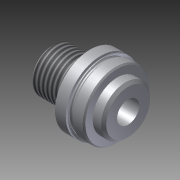
# Autodesk Inventor part: 04000_rod_guide
Saved by Autodesk Inventor 2012 (Build 160160000, 160)
## iProperties
Category: PARTsolutions
Company: BIMBA
Created: 2013-01-17
Part Number: 04000_rod_guide
Material: Default
Catalog Web Link: www.cadenas.de
Description: Rod Guide-Original Line - Standard Air Cylinders
Vendor: BIMBA
Document SubType Name: Modeling
Designer: William
Manufacturer: BIMBA
Density: 1 g/cm^3
Mass: 3.5706 g
Surface Area: 22.4703 cm^2
Volume: 3.5706 cm^3
PSOL_IDENT_0: {\\10.0.0.242\data_v9\23d-libs\bimba\bimba\bimba_imperial\bimba_full_line\original_line_cylinders\st
PSOL_IDENT_1: andard_air_cylinders\rod_guide.prj},217 {VTYP=3D},{NB=04000_rod_guide},{LINA=04000_rod_guide},{NN=Ro
PSOL_IDENT_2: d Guide},{DATE=11.09.2012 04:45:35},{GEOMDATE=11.09.2012 04:45:00},{VERSION=},{LINEID=40},{LINESUBID
PSOL_IDENT_3: =-1},{WBVAR=MNT,ACTING,NR,K,Q,T1,T2,T3,T4,MB,TRIM,CUSH}  {NB=04000_rod_guide},{LINA=04000_rod_guide}
PSOL_IDENT_4: ,{KT=DUMMY},{PN=04000},{BORE=0.75000000},{BOREPN=04},{MNT=},{MNTALG='' , 'Front Nose' , 'BF' , 'Fron
PSOL_IDENT_5: t Block' , 'BFT' , 'Front Trunnion' , 'A' , 'Adjustable Stroke'},{ACTING=},{ACTINGALG= '' , 'Single
PSOL_IDENT_6: Acting' , 'R' , 'Reverse/Double Acting' },{NR=},{NRALG= '' , 'Without Non-rotating Rod' , 'NR' , 'Wi
PSOL_IDENT_7: th Non-rotating Rod' },{K=},{Q=},{QALG= '' , 'Without Side Ported Rear Head' , 'Q' , 'With Side Port
PSOL_IDENT_8: ed Rear Head' },{T1=},{T2=},{T3=},{T4=},{MB=0},{A1=0.8750},{A1N=0.8750},{A1P=1.5940},{A1B=1.5940},{A
PSOL_IDENT_9: 2=0.4380},{A2N=0.4380},{A2P=0.5000},{A3=0.1240},{A3N=0.1240},{A3P=0.8440},{A4=0.3130},{A4N=0.3130},{
PSOL_IDENT_10: A4P=0.2525},{A5=0.0300},{A6=0.1250},{A6N=0.1250},{A6P=0.0000},{A7=0.4390},{A7N=0.4390},{A7P=0.2500},
PSOL_IDENT_11: {A8=0.0100},{A8N=0.0100},{A8NR=0.0300},{D1=0.8050},{D1N=0.8050},{D1P=0.8625},{D1B=0.8325},{D2=0.7615
PSOL_IDENT_12: },{D3=0.5620},{D3N=0.5620},{D3P=0.0000},{D4=0.2605},{D4N=0.2605},{D4P=0.5310},{D4NR=0.3120},{D5=0.25
PSOL_IDENT_13: 35},{D5N=0.2535},{D5NR=0.2515},{C1=0.030},{C2=0.0150},{C2N=0.0150},{C2P=0.0300},{C3=0.0000},{C3N=0.0
PSOL_IDENT_14: 000},{C3P=0.0000},{C4=0.0000},{C4N=0.0000},{C4P=0.0300},{NDM=0.5000},{NDMN=0.5000},{NDMP=0.6250},{TA
PSOL_IDENT_15: B=UNF},{D6=0.6225},{D6N=0.6225},{D6P=0.6225},{A9=0.0940},{A9N=0.0940},{A9P=0.0940},{D7=0.5385},{D7N=
PSOL_IDENT_16: 0.5385},{D7P=0.5385},{A10=0.0855},{A10N=0.0855},{A10P=0.0855},{R1=0.0345},{R1N=0.0345},{R1P=0.0345},
PSOL_IDENT_17: {D8=0.5310},{D9=0.5000},{D10=0.4405},{A11=0.8030},{A12=0.8970},{A13=1.0220},{A14=0.6250},{A14N=0.625
PSOL_IDENT_18: 0},{A14B=0.6250},{D11=0.2500},{D11N=0.2500},{NDM2=0.4050},{NDM2N=0.4050},{NDM2DP=0.2500},{THREAD=1},
PSOL_IDENT_19: {HEX=0.2535},{HEXN=0.2535},{S1=1.0000},{B1=0.1250},{B2=0.4690},{B22=0.0000},{DB=0.0000},{B3=0.3800},
PSOL_IDENT_20: {B4=0.6300},{X1=0.0920},{X2=0.6225},{NDM3=0.2500},{NDM4=0.1900},{NDM4DP=0.2500},{DD=1.0000},{CB=0.32
PSOL_IDENT_21: 80},{CBDP=0.2190},{PORT=1},{XT=0.4380},{XTX=0.4380},{XT1=0.5000},{XT2=0.5000},{NDMH=0.4375},{OD=0.80
PSOL_IDENT_22: 50},{ID=0.7615},{G=0.0000},{PNUT=0.4380},{TRIM=0},{C11=0.2380},{C22=0.2750},{C33=0.1950},{C44=0.3700
PSOL_IDENT_23: },{C55=0.5350},{CD1=0.1900},{CD2=0.1500},{CD3=0.0725},{CNDM3=0.1380},{CTAB3=UNF},{CUSH=0},{XX=0.6300
PSOL_IDENT_24: 0},{LCD=0.0000}
CNS_NT: Original Line - Standard Air Cylinders
CNS_NB: 04000_rod_guide
CNS_NBSYN: $PN._rod_guide
CNS_LINA: 04000_rod_guide
CNS_PN: 04000
CNS_BORE: 3/4
CNS_BOREPN: 04
CNS_MNT: Front Nose
CNS_MNTALG: '' , 'Front Nose' , 'BF' , 'Front Block' , 'BFT' , 'Front Trunnion' , 'A' , 'Adjustable Stroke'
CNS_ACTING: Single Acting
CNS_ACTINGALG: '' , 'Single Acting' , 'R' , 'Reverse/Double Acting'
CNS_NR: Without Non-rotating Rod
CNS_NRALG: '' , 'Without Non-rotating Rod' , 'NR' , 'With Non-rotating Rod'
CNS_K: Standard
CNS_Q: Without Side Ported Rear Head
CNS_QALG: '' , 'Without Side Ported Rear Head' , 'Q' , 'With Side Ported Rear Head'
CNS_T1: without T1
CNS_T2: without T2
CNS_T3: without T3
CNS_T4: without T4
CNS_MB: 0
CNS_A1: 0.8750
CNS_A1N: 0.8750
CNS_A1P: 1.5940
CNS_A1B: 1.5940
CNS_A2: 0.4380
CNS_A2N: 0.4380
CNS_A2P: 0.5000
CNS_A3: 0.1240
CNS_A3N: 0.1240
CNS_A3P: 0.8440
CNS_A4: 0.3130
CNS_A4N: 0.3130
CNS_A4P: 0.2525
CNS_A5: 0.0300
CNS_A6: 0.1250
CNS_A6N: 0.1250
CNS_A6P: 0.0000
CNS_A7: 0.4390
CNS_A7N: 0.4390
CNS_A7P: 0.2500
CNS_A8: 0.0100
CNS_A8N: 0.0100
CNS_A8NR: 0.0300
CNS_D1: 0.8050
CNS_D1N: 0.8050
CNS_D1P: 0.8625
CNS_D1B: 0.8325
CNS_D2: 0.7615
CNS_D3: 0.5620
CNS_D3N: 0.5620
CNS_D3P: 0.0000
CNS_D4: 0.2605
CNS_D4N: 0.2605
CNS_D4P: 0.5310
CNS_D4NR: 0.3120
CNS_D5: 0.2535
CNS_D5N: 0.2535
CNS_D5NR: 0.2515
CNS_C1: 0.030
CNS_C2: 0.0150
CNS_C2N: 0.0150
CNS_C2P: 0.0300
CNS_C3: 0.0000
CNS_C3N: 0.0000
CNS_C3P: 0.0000
CNS_C4: 0.0000
CNS_C4N: 0.0000
CNS_C4P: 0.0300
CNS_NDM: 0.5000
CNS_NDMN: 0.5000
CNS_NDMP: 0.6250
CNS_TAB: UNF
CNS_D6: 0.6225
CNS_D6N: 0.6225
CNS_D6P: 0.6225
CNS_A9: 0.0940
CNS_A9N: 0.0940
CNS_A9P: 0.0940
CNS_D7: 0.5385
CNS_D7N: 0.5385
CNS_D7P: 0.5385
CNS_A10: 0.0855
CNS_A10N: 0.0855
CNS_A10P: 0.0855
CNS_R1: 0.0345
CNS_R1N: 0.0345
CNS_R1P: 0.0345
CNS_D8: 0.5310
CNS_D9: 0.5000
CNS_D10: 0.4405
CNS_A11: 0.8030
CNS_A12: 0.8970
CNS_A13: 1.0220
CNS_A14: 0.6250
CNS_A14N: 0.6250
CNS_A14B: 0.6250
CNS_D11: 0.2500
CNS_D11N: 0.2500
CNS_NDM2: 0.4050
CNS_NDM2N: 0.4050
CNS_NDM2DP: 0.2500
CNS_THREAD: 1
CNS_HEX: 0.2535
CNS_HEXN: 0.2535
CNS_S1: 1.0000
CNS_B1: 0.1250
CNS_B2: 0.4690
CNS_B22: 0.0000
CNS_DB: 0.0000
CNS_B3: 0.3800
CNS_B4: 0.6300
CNS_X1: 0.0920
CNS_X2: 0.6225
CNS_NDM3: 0.2500
CNS_NDM4: 0.1900
CNS_NDM4DP: 0.2500
CNS_DD: 1.0000
CNS_CB: 0.3280
CNS_CBDP: 0.2190
CNS_PORT: 1
CNS_XT: 0.4380
CNS_XTX: 0.4380
CNS_XT1: 0.5000
CNS_XT2: 0.5000
CNS_NDMH: 0.4375
CNS_OD: 0.8050
CNS_ID: 0.7615
CNS_G: 0.0000
CNS_PNUT: 0.4380
CNS_TRIM: 0
CNS_C11: 0.2380
CNS_C22: 0.2750
CNS_C33: 0.1950
CNS_C44: 0.3700
CNS_C55: 0.5350
CNS_CD1: 0.1900
CNS_CD2: 0.1500
CNS_CD3: 0.0725
CNS_CNDM3: 0.1380
CNS_CTAB3: UNF
CNS_CUSH: 0
CNS_XX: 0.63000
CNS_LCD: 0.0000
SUPPLIER: BIMBA
ARTICLENO: 04000_rod_guide
BOMINFO: 04000_rod_guide
CREATOR: CADENAS GmbH
Title: 04000_rod_guide
Author: Cadenas PARTsolutions
Comments: Original Line - Standard Air Cylinders
Autodesk Inventor part; units mm, degrees
sketch "Sketch_1" plane through (0, 0, 0) normal (0, 0, 1) x (1, 0, 0)
  line L0 (11.1252, 0) -> (0, 0)
  line L1 (0, 0) -> (0, 5.5944)
  line L2 (0, 5.5944) -> (0.7557, 6.35)
  line L3 (0.7557, 6.35) -> (11.1252, 6.35)
  line L4 (11.1252, 6.35) -> (11.1252, 0)
  line L5 (11.1252, 0) -> (0, 0)
  constraints: 12 end point
revolve "Revolution1" add sketch "Sketch_1" angle 360 about axis through (11.1252, 0, 0) along (1, 0, 0)
thread "Thread1" size "1/2-20 UNF" class "2A" standard "ANSI Unified Screw Threads" full length
sketch "Sketch_3" plane through (0, 0, 0) normal (0, 0, 1) x (1, 0, 0)
  line L0 (19.05, 0) -> (11.1252, 0)
  line L1 (11.1252, 0) -> (11.1252, 10.2235)
  line L2 (11.1252, 10.2235) -> (14.2748, 10.2235)
  line L3 (14.2748, 10.2235) -> (14.2748, 8.9091)
  line L4 (14.2748, 8.9091) -> (15.0368, 8.9091)
  line L5 (15.0368, 8.9091) -> (15.7988, 9.671)
  line L6 (15.7988, 9.671) -> (18.669, 9.671)
  line L7 (18.669, 9.671) -> (19.05, 9.2901)
  line L8 (19.05, 9.2901) -> (19.05, 0)
  line L9 (19.05, 0) -> (11.1252, 0)
  constraints: 20 end point
revolve "Revolution2" add sketch "Sketch_3" angle 360 about axis through (19.05, 0, 0) along (1, 0, 0)
sketch "Sketch_4" plane through (0, 0, 0) normal (0, 0, 1) x (1, 0, 0)
  line L0 (22.225, 0) -> (19.05, 0)
  line L1 (19.05, 0) -> (19.05, 7.1374)
  line L2 (19.05, 7.1374) -> (21.463, 7.1374)
  line L3 (21.463, 7.1374) -> (22.225, 6.3754)
  line L4 (22.225, 6.3754) -> (22.225, 0)
  line L5 (22.225, 0) -> (19.05, 0)
  constraints: 12 end point
revolve "Revolution3" add sketch "Sketch_4" angle 360 about axis through (22.225, 0, 0) along (1, 0, 0)
sketch "Sketch4" plane through (0, 0, 0) normal (-1, 0, 0) x (0, 0, 1)
  point P0 (0, 0)
hole "Drilling 1" at (0, 0, 0) direction (1, 0, 0) diameter 6.4389 depth 22.225 countersink diameter 6.9469 countersink angle 90
sketch "Sketch_47" plane through (0, 0, 0) normal (0, 0, 1) x (1, 0, 0)
  line L0 (15.0368, 0) -> (14.2748, 0)
  line L1 (14.2748, 8.655) -> (15.0368, 8.655)
  line L2 (15.0368, 8.655) -> (15.0368, 8.9091)
  line L3 (15.0368, 8.9091) -> (14.6558, 8.9091)
  line L4 (14.6558, 8.9091) -> (14.3973, 9.1676)
  arc A0 (14.3973, 9.3472) -> (14.3973, 9.1676) centre (14.4871, 9.2574) ccw
  line L5 (14.3973, 9.3472) -> (15.1895, 10.1393)
  line L6 (15.1895, 10.1393) -> (15.1895, 10.2235)
  line L7 (15.1895, 10.2235) -> (14.9863, 10.2235)
  line L8 (14.9863, 10.2235) -> (14.2748, 9.512)
  line L9 (14.2748, 9.512) -> (14.2748, 8.655)
  constraints: 20 end point, 2 point on circle, 1 centre point
revolve "Revolution4" add sketch "Sketch_47" angle 360 about axis through (15.0368, 0, 0) along (1, 0, 0)
ref_plane "rod_guide_XY" through (0, 0, 0) normal (1, 0, 0) x (0, 0, -1)
ref_plane "rod_guide_YZ" through (0, 0, 0) normal (0, 0, -1) x (0, 1, 0)
ref_plane "rod_guide_ZX" through (0, 0, 0) normal (0, 1, 0) x (1, 0, 0)
ref_plane "to_tube_XY" through (15.0368, 0, 0) normal (1, 0, 0) x (0, 0, -1)
ref_plane "to_tube_YZ" through (15.0368, 0, 0) normal (0, 0, -1) x (0, 1, 0)
ref_plane "to_tube_ZX" through (15.0368, 0, 0) normal (0, 1, 0) x (1, 0, 0)
ref_plane "to_foot_bracket_XY" through (11.1252, 0, 0) normal (1, 0, 0) x (0, 0, -1)
ref_plane "to_foot_bracket_YZ" through (11.1252, 0, 0) normal (0, 0, -1) x (0, 1, 0)
ref_plane "to_foot_bracket_ZX" through (11.1252, 0, 0) normal (0, 1, 0) x (1, 0, 0)
ref_plane "to_nut_XY" through (11.1252, 0, 0) normal (1, 0, 0) x (0, 0, -1)
ref_plane "to_nut_YZ" through (11.1252, 0, 0) normal (0, 0, -1) x (0, 1, 0)
ref_plane "to_nut_ZX" through (11.1252, 0, 0) normal (0, 1, 0) x (1, 0, 0)
ref_plane "to_trunnion_brackets_XY" through (11.1252, 0, 0) normal (0, 1, 0) x (1, 0, 0)
ref_plane "to_trunnion_brackets_YZ" through (11.1252, 0, 0) normal (1, 0, 0) x (0, 0, -1)
ref_plane "to_trunnion_brackets_ZX" through (11.1252, 0, 0) normal (0, 0, -1) x (0, 1, 0)
ref_plane "to_trunnion_brackets1_XY" through (11.1252, 12.7, 0) normal (0, 1, 0) x (1, 0, 0)
ref_plane "to_trunnion_brackets1_YZ" through (11.1252, 12.7, 0) normal (1, 0, 0) x (0, 0, -1)
ref_plane "to_trunnion_brackets1_ZX" through (11.1252, 12.7, 0) normal (0, 0, -1) x (0, 1, 0)
ref_plane "to_trunnion_brackets2_XY" through (11.1252, -12.7, 0) normal (0, 1, 0) x (1, 0, 0)
ref_plane "to_trunnion_brackets2_YZ" through (11.1252, -12.7, 0) normal (1, 0, 0) x (0, 0, -1)
ref_plane "to_trunnion_brackets2_ZX" through (11.1252, -12.7, 0) normal (0, 0, -1) x (0, 1, 0)
ref_plane "t111_XY" through (11.1252, 0, 0) normal (1, 0, 0) x (0, 0, -1)
ref_plane "t111_YZ" through (11.1252, 0, 0) normal (0, 0, -1) x (0, 1, 0)
ref_plane "t111_ZX" through (11.1252, 0, 0) normal (0, 1, 0) x (1, 0, 0)
ref_plane "t1_XY" through (11.1252, 0, 0) normal (1, 0, 0) x (0, 0, -1)
ref_plane "t1_YZ" through (11.1252, 0, 0) normal (0, 0, -1) x (0, 1, 0)
ref_plane "t1_ZX" through (11.1252, 0, 0) normal (0, 1, 0) x (1, 0, 0)
ref_plane "to_screw_XY" through (6.35, 2.032, -6.0452) normal (0, 1, 0) x (1, 0, 0)
ref_plane "to_screw_YZ" through (6.35, 2.032, -6.0452) normal (1, 0, 0) x (0, 0, -1)
ref_plane "to_screw_ZX" through (6.35, 2.032, -6.0452) normal (0, 0, -1) x (0, 1, 0)
body "Solid1"
